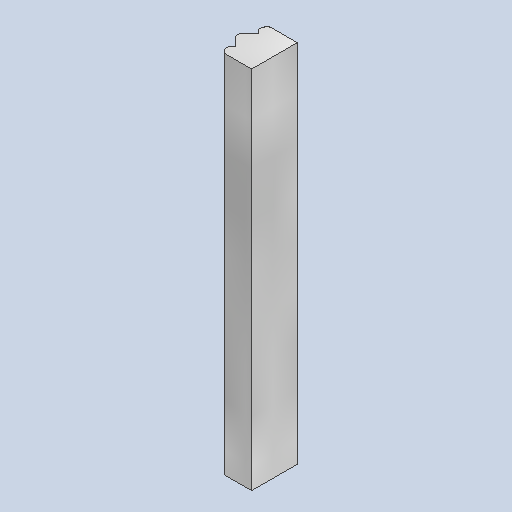
# Autodesk Inventor part: 窗間柱
Saved by Autodesk Inventor 2024.2 (Build 282272000, 272)
## iProperties
Created: 2024-05-31
Part Number: 窗間柱
Material: 一般
Document SubType Name: Modeling
Designer: User
Density: 1 g/cm^3
Appearance: 預設
Author: User
Autodesk Inventor part; units mm, degrees
ref_plane "YZ Plane" through (0, 0, 0) normal (1, 0, 0) x (0, 1, 0)
ref_plane "XZ Plane" through (0, 0, 0) normal (0, 1, 0) x (-1, 0, 0)
ref_plane "XY Plane" through (0, 0, 0) normal (0, 0, 1) x (1, 0, 0)
sketch "草圖1" plane through (0, 0, 0) normal (0, 1, 0) x (-1, 0, 0)
  line L0 (-0.3, 0.5) -> (-0.3, -0.5)
  line L1 (-0.3, -0.5) -> (0.3, -0.5)
  line L2 (0.3, -0.5) -> (0.3, 0.5)
  line L3 (0.3, 0.5) -> (-0.3, 0.5)
  line L4 (-0.3, 0.5) -> (0.3, -0.5) construction
  line L5 (-0.3, -0.5) -> (0.3, 0.5) construction
  line L6 (0.3, 0.5) -> (0.3, 0.25)
  line L7 (0.3, 0.25) -> (0.3, -0.25)
  line L8 (0.3, -0.25) -> (0.3, -0.5)
  line L9 (0.3, 0.25) -> (0.55, 0)
  line L10 (0.55, 0) -> (0.3, -0.25)
  line L11 (0.3, -0.25) -> (0.425, -0.375)
  line L12 (0.425, -0.375) -> (0.3, -0.5)
  line L13 (0.3, 0.25) -> (0.425, 0.375)
  line L14 (0.425, 0.375) -> (0.3, 0.5)
  point P0 (0, 0)
  dimension "d0" = 1
  dimension "d1" = 0.6
  dimension "d2" = 0.25
  dimension "d3" = 0.5
  dimension "d4" = 45
  constraints: 30 end point, 5 perpendicular, 3 parallel, 3 point on line, 2 midpoint, 1 collinear, 1 vertical
  measures "d0" distance of L0.start L0.end
  measures "d1" distance of L1.end L0.end
  measures "d2" distance of L2.end L6.end
  measures "d3" distance of L6.end L7.end
  measures "d4" angle of L10 L2
extrude "擠出1" add sketch "草圖1" along normal blind 8
fillet "圓角1" radius 0.1 3 edges at (-0.55, 4, 0) (-0.425, 4, -0.375) (-0.425, 4, 0.375)
